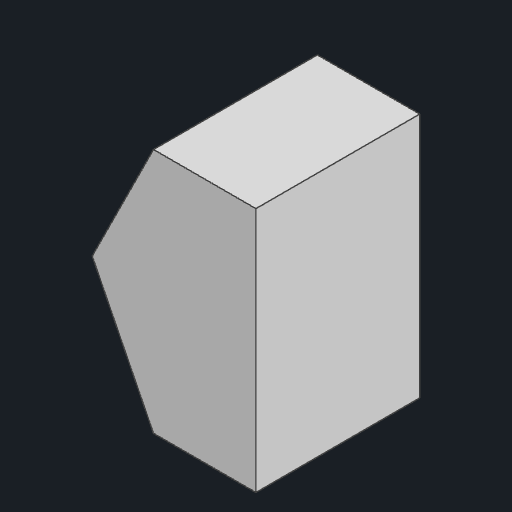
# Autodesk Inventor part: hand
Saved by Autodesk Inventor 2023 (Build 270158000, 158)
## iProperties
Created: 2024-02-21
Part Number: hand
Material: Generic
Document SubType Name: Modeling
Designer: valer
Density: 1 g/cm^3
Appearance: Default
Author: valer
Autodesk Inventor part; units mm, degrees
ref_plane "YZ Plane" through (0, 0, 0) normal (1, 0, 0) x (0, 1, 0)
ref_plane "XZ Plane" through (0, 0, 0) normal (0, 1, 0) x (-1, 0, 0)
ref_plane "XY Plane" through (0, 0, 0) normal (0, 0, 1) x (1, 0, 0)
sketch "Sketch1" plane through (0, 0, 0) normal (0, 0, 1) x (1, 0, 0)
  line L0 (-100, 0) -> (-25.2128, 150)
  line L1 (-25.2128, 150) -> (99.7872, 150)
  line L2 (99.7872, 150) -> (99.7872, 0)
  line L3 (99.7872, 0) -> (-100, 0) construction
  line L4 (-100, 0) -> (-25.2128, -150)
  line L5 (-25.2128, -150) -> (99.7872, -150)
  line L6 (99.7872, -150) -> (99.7872, 0)
  line L7 (-139.9574, 0) -> (139.7447, 0) projected
  point P0 (0, 0)
  dimension "d0" = 127
  dimension "d1" = 125
  dimension "d4" = 300
  dimension "d5" = 100
  constraints: 14 end point, 2 perpendicular, 2 symmetric about line, 1 coincident, 1 horizontal, 1 point on line
  measures "d0" angle of L4 L0
  measures "d1" distance of L0.end L1.end
  measures "d4" distance between parallel lines of L5 L1
  measures "d5" distance of point (0, 0) point (-100, 0)
extrude "Extrusion1" add sketch "Sketch1" along normal mid plane 200
body "Solid1"
